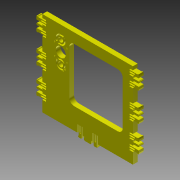
# Autodesk Inventor part: sideB
Saved by Autodesk Inventor 2012 SP1 (Build 160190100, 190)
## iProperties
Created: 2011-10-14
Part Number: sideB
Document SubType Name: Modeling
Designer: cramera
Density: 0.952 g/cm^3
Material: High Density Polyethylene
Mass: 347.048 g
Surface Area: 1035.52 cm^2
Volume: 364.546 cm^3
Autodesk Inventor part; units mm, degrees
ref_plane "YZ Plane" through (0, 0, 0) normal (1, 0, 0) x (0, 1, 0)
ref_plane "XZ Plane" through (0, 0, 0) normal (0, 1, 0) x (-1, 0, 0)
ref_plane "XY Plane" through (0, 0, 0) normal (0, 0, 1) x (1, 0, 0)
derived "skeleton.ipt"
sketch "DRILL-THROUGH" plane through (0, 0, 0) normal (0, 0, 1) x (1, 0, 0)
  arc A0 (221.6732, 527.9859) -> (220.0857, 526.3984) centre (221.6732, 526.3984) ccw
  arc A1 (220.0857, 526.3984) -> (221.6732, 524.8109) centre (221.6732, 526.3984) ccw
  arc A2 (221.6732, 524.8109) -> (223.2607, 526.3984) centre (221.6732, 526.3984) ccw
  arc A3 (223.2607, 526.3984) -> (221.6732, 527.9859) centre (221.6732, 526.3984) ccw
  arc A4 (252.6612, 527.9859) -> (251.0737, 526.3984) centre (252.6612, 526.3984) ccw
  arc A5 (251.0737, 526.3984) -> (252.6612, 524.8109) centre (252.6612, 526.3984) ccw
  arc A6 (252.6612, 524.8109) -> (254.2487, 526.3984) centre (252.6612, 526.3984) ccw
  arc A7 (254.2487, 526.3984) -> (252.6612, 527.9859) centre (252.6612, 526.3984) ccw
  arc A8 (252.6612, 496.9979) -> (251.0737, 495.4104) centre (252.6612, 495.4104) ccw
  arc A9 (251.0737, 495.4104) -> (252.6612, 493.8229) centre (252.6612, 495.4104) ccw
  arc A10 (252.6612, 493.8229) -> (254.2487, 495.4104) centre (252.6612, 495.4104) ccw
  arc A11 (254.2487, 495.4104) -> (252.6612, 496.9979) centre (252.6612, 495.4104) ccw
  arc A12 (221.6732, 496.9979) -> (220.0857, 495.4104) centre (221.6732, 495.4104) ccw
  arc A13 (220.0857, 495.4104) -> (221.6732, 493.8229) centre (221.6732, 495.4104) ccw
  arc A14 (221.6732, 493.8229) -> (223.2607, 495.4104) centre (221.6732, 495.4104) ccw
  arc A15 (223.2607, 495.4104) -> (221.6732, 496.9979) centre (221.6732, 495.4104) ccw
  constraints: 32 point on circle, 16 centre point
sketch "POCKET_1-8" plane through (0, 0, 0) normal (0, 0, 1) x (1, 0, 0)
  arc A0 (256.4712, 495.4104) -> (252.6612, 499.2204) centre (252.6612, 495.4104) ccw
  arc A1 (221.6732, 499.2204) -> (217.8632, 495.4104) centre (221.6732, 495.4104) ccw
  arc A2 (217.8632, 495.4104) -> (221.6732, 491.6004) centre (221.6732, 495.4104) ccw
  arc A3 (221.6732, 491.6004) -> (225.4832, 495.4104) centre (221.6732, 495.4104) ccw
  arc A4 (225.4832, 495.4104) -> (221.6732, 499.2204) centre (221.6732, 495.4104) ccw
  arc A5 (252.6612, 530.2084) -> (248.8512, 526.3984) centre (252.6612, 526.3984) ccw
  arc A6 (248.8512, 526.3984) -> (252.6612, 522.5884) centre (252.6612, 526.3984) ccw
  arc A7 (252.6612, 522.5884) -> (256.4712, 526.3984) centre (252.6612, 526.3984) ccw
  arc A8 (256.4712, 526.3984) -> (252.6612, 530.2084) centre (252.6612, 526.3984) ccw
  arc A9 (221.6732, 530.2084) -> (217.8632, 526.3984) centre (221.6732, 526.3984) ccw
  arc A10 (217.8632, 526.3984) -> (221.6732, 522.5884) centre (221.6732, 526.3984) ccw
  arc A11 (221.6732, 522.5884) -> (225.4832, 526.3984) centre (221.6732, 526.3984) ccw
  arc A12 (225.4832, 526.3984) -> (221.6732, 530.2084) centre (221.6732, 526.3984) ccw
  arc A13 (252.6612, 499.2204) -> (248.8512, 495.4104) centre (252.6612, 495.4104) ccw
  arc A14 (248.8512, 495.4104) -> (252.6612, 491.6004) centre (252.6612, 495.4104) ccw
  arc A15 (252.6612, 491.6004) -> (256.4712, 495.4104) centre (252.6612, 495.4104) ccw
  constraints: 32 point on circle, 16 centre point
sketch "STOCK_12MM" plane through (0, 0, 0) normal (0, 0, 1) x (1, 0, 0)
  line L0 (457.2, 0) -> (457.2, 914.4)
  line L1 (457.2, 914.4) -> (0, 914.4)
  line L2 (0, 914.4) -> (0, 0)
  line L3 (457.2, 914.4) -> (457.2, 0)
  line L4 (0, 0) -> (457.2, 0)
  constraints: 10 end point
sketch "THROUGH-CUT" plane through (0, 0, 0) normal (0, 0, 1) x (1, 0, 0)
  line L0 (271.4572, 409.3044) -> (381.6297, 409.3044)
  arc A0 (381.6297, 409.3044) -> (394.3297, 422.0044) centre (381.6297, 422.0044) ccw
  line L1 (394.3297, 422.0044) -> (394.3297, 533.1294)
  arc A1 (394.3297, 533.1294) -> (381.6297, 545.8294) centre (381.6297, 533.1294) ccw
  line L2 (381.6297, 545.8294) -> (271.4572, 545.8294)
  arc A2 (271.4572, 545.8294) -> (258.7572, 533.1294) centre (271.4572, 533.1294) ccw
  line L3 (258.7572, 533.1294) -> (258.7572, 422.0044)
  arc A3 (258.7572, 422.0044) -> (271.4572, 409.3044) centre (271.4572, 422.0044) ccw
  circle A4 centre (237.1672, 510.9044) radius 12.7
  circle A5 centre (237.1672, 537.8919) radius 5.925
  circle A6 centre (237.1672, 483.9169) radius 5.925
  arc A7 (410.2047, 390.0639) -> (411.7922, 388.4764) centre (411.7922, 390.0639) ccw
  line L4 (410.2047, 390.0639) -> (410.2047, 390.1909)
  arc A8 (411.7922, 391.7784) -> (410.2047, 390.1909) centre (411.7922, 390.1909) ccw
  line L5 (411.7922, 391.7784) -> (423.3207, 391.7784)
  arc A9 (424.9082, 390.1909) -> (423.3207, 391.7784) centre (423.3207, 390.1909) ccw
  line L6 (424.9082, 390.1909) -> (424.9082, 390.0639)
  arc A10 (423.3207, 388.4764) -> (424.9082, 390.0639) centre (423.3207, 390.0639) ccw
  line L7 (423.3207, 388.4764) -> (411.7922, 388.4764)
  arc A11 (423.3207, 553.8304) -> (424.9082, 555.4179) centre (423.3207, 555.4179) ccw
  line L8 (424.9082, 555.4179) -> (424.9082, 555.5449)
  arc A12 (424.9082, 555.5449) -> (423.3207, 557.1324) centre (423.3207, 555.5449) ccw
  line L9 (423.3207, 557.1324) -> (411.7922, 557.1324)
  arc A13 (411.7922, 557.1324) -> (410.2047, 555.5449) centre (411.7922, 555.5449) ccw
  line L10 (410.2047, 555.5449) -> (410.2047, 555.4179)
  arc A14 (410.2047, 555.4179) -> (411.7922, 553.8304) centre (411.7922, 555.4179) ccw
  line L11 (411.7922, 553.8304) -> (423.3207, 553.8304)
  arc A15 (410.2047, 415.7179) -> (411.7922, 414.1304) centre (411.7922, 415.7179) ccw
  line L12 (411.7922, 414.1304) -> (423.3207, 414.1304)
  arc A16 (423.3207, 414.1304) -> (424.9082, 415.7179) centre (423.3207, 415.7179) ccw
  line L13 (424.9082, 415.7179) -> (424.9082, 415.8449)
  arc A17 (424.9082, 415.8449) -> (423.3207, 417.4324) centre (423.3207, 415.8449) ccw
  line L14 (423.3207, 417.4324) -> (411.7922, 417.4324)
  arc A18 (411.7922, 417.4324) -> (410.2047, 415.8449) centre (411.7922, 415.8449) ccw
  line L15 (410.2047, 415.8449) -> (410.2047, 415.7179)
  arc A19 (423.3207, 455.1514) -> (424.9082, 456.7389) centre (423.3207, 456.7389) ccw
  line L16 (423.3207, 455.1514) -> (411.7922, 455.1514)
  arc A20 (410.2047, 456.7389) -> (411.7922, 455.1514) centre (411.7922, 456.7389) ccw
  line L17 (410.2047, 456.7389) -> (410.2047, 456.8659)
  arc A21 (411.7922, 458.4534) -> (410.2047, 456.8659) centre (411.7922, 456.8659) ccw
  line L18 (411.7922, 458.4534) -> (423.3207, 458.4534)
  arc A22 (424.9082, 456.8659) -> (423.3207, 458.4534) centre (423.3207, 456.8659) ccw
  line L19 (424.9082, 456.8659) -> (424.9082, 456.7389)
  arc A23 (423.3207, 528.1764) -> (424.9082, 529.7639) centre (423.3207, 529.7639) ccw
  line L20 (423.3207, 528.1764) -> (411.7922, 528.1764)
  arc A24 (410.2047, 529.7639) -> (411.7922, 528.1764) centre (411.7922, 529.7639) ccw
  line L21 (410.2047, 529.7639) -> (410.2047, 529.8909)
  arc A25 (411.7922, 531.4784) -> (410.2047, 529.8909) centre (411.7922, 529.8909) ccw
  line L22 (411.7922, 531.4784) -> (423.3207, 531.4784)
  arc A26 (424.9082, 529.8909) -> (423.3207, 531.4784) centre (423.3207, 529.8909) ccw
  line L23 (424.9082, 529.8909) -> (424.9082, 529.7639)
  arc A27 (284.6017, 358.0885) -> (286.1892, 356.501) centre (286.1892, 358.0885) ccw
  line L24 (284.6017, 358.0885) -> (284.6017, 372.7919)
  arc A28 (286.1892, 374.3794) -> (284.6017, 372.7919) centre (286.1892, 372.7919) ccw
  line L25 (286.1892, 374.3794) -> (286.3162, 374.3794)
  arc A29 (287.9037, 372.7919) -> (286.3162, 374.3794) centre (286.3162, 372.7919) ccw
  line L26 (287.9037, 372.7919) -> (287.9037, 358.0885)
  arc A30 (286.3162, 356.501) -> (287.9037, 358.0885) centre (286.3162, 358.0885) ccw
  line L27 (286.3162, 356.501) -> (286.1892, 356.501)
  arc A31 (187.5388, 417.4324) -> (185.9513, 415.8449) centre (187.5388, 415.8449) ccw
  line L28 (187.5388, 417.4324) -> (199.0672, 417.4324)
  arc A32 (200.6547, 415.8449) -> (199.0672, 417.4324) centre (199.0672, 415.8449) ccw
  line L29 (200.6547, 415.8449) -> (200.6547, 415.7179)
  arc A33 (199.0672, 414.1304) -> (200.6547, 415.7179) centre (199.0672, 415.7179) ccw
  line L30 (199.0672, 414.1304) -> (187.5388, 414.1304)
  arc A34 (185.9513, 415.7179) -> (187.5388, 414.1304) centre (187.5388, 415.7179) ccw
  line L31 (185.9513, 415.7179) -> (185.9513, 415.8449)
  arc A35 (187.5388, 391.7784) -> (185.9513, 390.1909) centre (187.5388, 390.1909) ccw
  line L32 (185.9513, 390.1909) -> (185.9513, 390.0639)
  arc A36 (185.9513, 390.0639) -> (187.5388, 388.4764) centre (187.5388, 390.0639) ccw
  line L33 (187.5388, 388.4764) -> (199.0672, 388.4764)
  arc A37 (199.0672, 388.4764) -> (200.6547, 390.0639) centre (199.0672, 390.0639) ccw
  line L34 (200.6547, 390.0639) -> (200.6547, 390.1909)
  arc A38 (200.6547, 390.1909) -> (199.0672, 391.7784) centre (199.0672, 390.1909) ccw
  line L35 (199.0672, 391.7784) -> (187.5388, 391.7784)
  arc A39 (199.0672, 480.8054) -> (200.6547, 482.3929) centre (199.0672, 482.3929) ccw
  line L36 (199.0672, 480.8054) -> (187.5388, 480.8054)
  arc A40 (185.9513, 482.3929) -> (187.5388, 480.8054) centre (187.5388, 482.3929) ccw
  line L37 (185.9513, 482.3929) -> (185.9513, 482.5199)
  arc A41 (187.5388, 484.1074) -> (185.9513, 482.5199) centre (187.5388, 482.5199) ccw
  line L38 (187.5388, 484.1074) -> (199.0672, 484.1074)
  arc A42 (200.6547, 482.5199) -> (199.0672, 484.1074) centre (199.0672, 482.5199) ccw
  line L39 (200.6547, 482.5199) -> (200.6547, 482.3929)
  arc A43 (228.9556, 532.1229) -> (229.2542, 533.9529) centre (227.8331, 533.2454) ccw
  line L40 (228.9556, 532.1229) -> (227.4719, 530.6392)
  arc A44 (225.2268, 530.6392) -> (227.4719, 530.6392) centre (226.3494, 531.7617) ccw
  line L41 (225.2268, 530.6392) -> (225.155, 530.711)
  arc A45 (225.155, 532.9561) -> (225.155, 530.711) centre (226.2775, 531.8336) ccw
  line L42 (225.155, 532.9561) -> (225.8266, 533.6277)
  arc A46 (241.4314, 549.2325) -> (225.8266, 533.6277) centre (237.1672, 537.8919) ccw
  line L43 (241.4314, 549.2325) -> (242.103, 549.9041)
  arc A47 (244.3481, 549.9041) -> (242.103, 549.9041) centre (243.2256, 548.7816) ccw
  line L44 (244.3481, 549.9041) -> (244.4199, 549.8323)
  arc A48 (244.4199, 547.5872) -> (244.4199, 549.8323) centre (243.2974, 548.7098) ccw
  line L45 (244.4199, 547.5872) -> (242.9362, 546.1035)
  arc A49 (241.1063, 545.8049) -> (242.9362, 546.1035) centre (241.8137, 547.226) ccw
  arc A50 (241.1063, 545.8049) -> (229.2542, 533.9529) centre (237.1672, 537.8919) ccw
  arc A51 (322.9557, 358.0885) -> (324.5432, 356.501) centre (324.5432, 358.0885) ccw
  line L46 (324.5432, 356.501) -> (324.6702, 356.501)
  arc A52 (324.6702, 356.501) -> (326.2577, 358.0885) centre (324.6702, 358.0885) ccw
  line L47 (326.2577, 358.0885) -> (326.2577, 372.7919)
  arc A53 (326.2577, 372.7919) -> (324.6702, 374.3794) centre (324.6702, 372.7919) ccw
  line L48 (324.6702, 374.3794) -> (324.5432, 374.3794)
  arc A54 (324.5432, 374.3794) -> (322.9557, 372.7919) centre (324.5432, 372.7919) ccw
  line L49 (322.9557, 372.7919) -> (322.9557, 358.0885)
  arc A55 (248.5078, 479.6527) -> (232.9031, 495.2575) centre (237.1672, 483.9169) ccw
  line L50 (232.9031, 495.2575) -> (232.2314, 495.9291)
  arc A56 (232.2314, 495.9291) -> (229.9864, 495.9291) centre (231.1089, 494.8066) ccw
  line L51 (229.9864, 495.9291) -> (229.9145, 495.8573)
  arc A57 (229.9145, 495.8573) -> (229.9145, 493.6122) centre (231.0371, 494.7348) ccw
  line L52 (229.9145, 493.6122) -> (231.3982, 492.1285)
  arc A58 (231.3982, 492.1285) -> (233.2282, 491.8299) centre (232.5208, 493.251) ccw
  arc A59 (245.0802, 479.9779) -> (233.2282, 491.8299) centre (237.1672, 483.9169) ccw
  arc A60 (245.0802, 479.9779) -> (245.3789, 478.1479) centre (246.5014, 479.2704) ccw
  line L53 (245.3789, 478.1479) -> (246.8626, 476.6642)
  arc A61 (246.8626, 476.6642) -> (249.1076, 476.6642) centre (247.9851, 477.7867) ccw
  line L54 (249.1076, 476.6642) -> (249.1795, 476.736)
  arc A62 (249.1795, 476.736) -> (249.1795, 478.9811) centre (248.0569, 477.8586) ccw
  line L55 (249.1795, 478.9811) -> (248.5078, 479.6527)
  arc A63 (199.0672, 528.1764) -> (200.6547, 529.7639) centre (199.0672, 529.7639) ccw
  line L56 (200.6547, 529.7639) -> (200.6547, 529.8909)
  arc A64 (200.6547, 529.8909) -> (199.0672, 531.4784) centre (199.0672, 529.8909) ccw
  line L57 (199.0672, 531.4784) -> (187.5388, 531.4784)
  arc A65 (187.5388, 531.4784) -> (185.9513, 529.8909) centre (187.5388, 529.8909) ccw
  line L58 (185.9513, 529.8909) -> (185.9513, 529.7639)
  arc A66 (185.9513, 529.7639) -> (187.5388, 528.1764) centre (187.5388, 529.7639) ccw
  line L59 (187.5388, 528.1764) -> (199.0672, 528.1764)
  arc A67 (423.3207, 480.8054) -> (424.9082, 482.3929) centre (423.3207, 482.3929) ccw
  line L60 (424.9082, 482.3929) -> (424.9082, 482.5199)
  arc A68 (424.9082, 482.5199) -> (423.3207, 484.1074) centre (423.3207, 482.5199) ccw
  line L61 (423.3207, 484.1074) -> (411.7922, 484.1074)
  arc A69 (411.7922, 484.1074) -> (410.2047, 482.5199) centre (411.7922, 482.5199) ccw
  line L62 (410.2047, 482.5199) -> (410.2047, 482.3929)
  arc A70 (410.2047, 482.3929) -> (411.7922, 480.8054) centre (411.7922, 482.3929) ccw
  line L63 (411.7922, 480.8054) -> (423.3207, 480.8054)
  arc A71 (187.5388, 458.4534) -> (185.9513, 456.8659) centre (187.5388, 456.8659) ccw
  line L64 (185.9513, 456.8659) -> (185.9513, 456.7389)
  arc A72 (185.9513, 456.7389) -> (187.5388, 455.1514) centre (187.5388, 456.7389) ccw
  line L65 (187.5388, 455.1514) -> (199.0616, 455.1514)
  arc A73 (199.0616, 455.1514) -> (200.6491, 456.7389) centre (199.0616, 456.7389) ccw
  line L66 (200.6491, 456.7389) -> (200.6547, 456.8659)
  arc A74 (200.6547, 456.8659) -> (199.0672, 458.4534) centre (199.0672, 456.8659) ccw
  line L67 (199.0672, 458.4534) -> (187.5388, 458.4534)
  arc A75 (225.8266, 488.1811) -> (241.4314, 472.5763) centre (237.1672, 483.9169) ccw
  line L68 (241.4314, 472.5763) -> (242.103, 471.9047)
  arc A76 (242.103, 471.9047) -> (244.3481, 471.9047) centre (243.2256, 473.0272) ccw
  line L69 (244.3481, 471.9047) -> (244.4199, 471.9765)
  arc A77 (244.4199, 471.9765) -> (244.4199, 474.2216) centre (243.2974, 473.099) ccw
  line L70 (244.4199, 474.2216) -> (242.9362, 475.7053)
  arc A78 (242.9362, 475.7053) -> (241.1063, 476.0039) centre (241.8137, 474.5827) ccw
  arc A79 (229.2542, 487.8559) -> (241.1063, 476.0039) centre (237.1672, 483.9169) ccw
  arc A80 (229.2542, 487.8559) -> (228.9556, 489.6859) centre (227.8331, 488.5634) ccw
  line L71 (228.9556, 489.6859) -> (227.4719, 491.1696)
  arc A81 (227.4719, 491.1696) -> (225.2268, 491.1696) centre (226.3494, 490.0471) ccw
  line L72 (225.2268, 491.1696) -> (225.155, 491.0978)
  arc A82 (225.155, 491.0978) -> (225.155, 488.8527) centre (226.2775, 489.9752) ccw
  line L73 (225.155, 488.8527) -> (225.8266, 488.1811)
  arc A83 (199.0672, 553.8304) -> (200.6547, 555.4179) centre (199.0672, 555.4179) ccw
  line L74 (199.0672, 553.8304) -> (187.5388, 553.8304)
  arc A84 (185.9513, 555.4179) -> (187.5388, 553.8304) centre (187.5388, 555.4179) ccw
  line L75 (185.9513, 555.4179) -> (185.9513, 555.5449)
  arc A85 (187.5388, 557.1324) -> (185.9513, 555.5449) centre (187.5388, 555.5449) ccw
  line L76 (187.5388, 557.1324) -> (199.0672, 557.1324)
  arc A86 (200.6547, 555.5449) -> (199.0672, 557.1324) centre (199.0672, 555.5449) ccw
  line L77 (200.6547, 555.5449) -> (200.6547, 555.4179)
  arc A87 (232.9031, 526.5513) -> (248.5078, 542.1561) centre (237.1672, 537.8919) ccw
  line L78 (232.9031, 526.5513) -> (232.2314, 525.8797)
  arc A88 (229.9864, 525.8797) -> (232.2314, 525.8797) centre (231.1089, 527.0022) ccw
  line L79 (229.9864, 525.8797) -> (229.9145, 525.9515)
  arc A89 (229.9145, 528.1966) -> (229.9145, 525.9515) centre (231.0371, 527.074) ccw
  line L80 (229.9145, 528.1966) -> (231.3982, 529.6803)
  arc A90 (233.2282, 529.9789) -> (231.3982, 529.6803) centre (232.5208, 528.5577) ccw
  arc A91 (233.2282, 529.9789) -> (245.0802, 541.8309) centre (237.1672, 537.8919) ccw
  arc A92 (245.3789, 543.6609) -> (245.0802, 541.8309) centre (246.5014, 542.5384) ccw
  line L81 (245.3789, 543.6609) -> (246.8626, 545.1446)
  arc A93 (249.1076, 545.1446) -> (246.8626, 545.1446) centre (247.9851, 544.0221) ccw
  line L82 (249.1076, 545.1446) -> (249.1795, 545.0728)
  arc A94 (249.1795, 542.8277) -> (249.1795, 545.0728) centre (248.0569, 543.9502) ccw
  line L83 (249.1795, 542.8277) -> (248.5078, 542.1561)
  arc A95 (288.3482, 346.4394) -> (289.9357, 348.0269) centre (288.3482, 348.0269) ccw
  line L84 (289.9357, 348.0269) -> (289.9357, 372.7919)
  arc A96 (291.5232, 374.3794) -> (289.9357, 372.7919) centre (291.5232, 372.7919) ccw
  line L85 (291.5232, 374.3794) -> (291.6502, 374.3794)
  arc A97 (293.2377, 372.7919) -> (291.6502, 374.3794) centre (291.6502, 372.7919) ccw
  line L86 (293.2377, 372.7919) -> (293.2377, 355.3294)
  line L87 (293.2377, 355.3294) -> (294.2947, 355.3294)
  arc A98 (296.5397, 353.0843) -> (294.2947, 355.3294) centre (295.4172, 354.2069) ccw
  line L88 (296.5397, 353.0843) -> (296.5397, 348.0269)
  line L89 (296.5397, 348.0269) -> (298.1272, 346.4394)
  line L90 (298.1272, 346.4394) -> (312.7322, 346.4394)
  line L91 (312.7322, 346.4394) -> (314.3197, 348.0269)
  line L92 (314.3197, 348.0269) -> (314.3197, 353.0843)
  arc A99 (316.5648, 355.3294) -> (314.3197, 353.0843) centre (315.4423, 354.2069) ccw
  line L93 (316.5648, 355.3294) -> (317.6217, 355.3294)
  line L94 (317.6217, 355.3294) -> (317.6217, 372.7919)
  arc A100 (319.2092, 374.3794) -> (317.6217, 372.7919) centre (319.2092, 372.7919) ccw
  line L95 (319.2092, 374.3794) -> (319.3362, 374.3794)
  arc A101 (320.9237, 372.7919) -> (319.3362, 374.3794) centre (319.3362, 372.7919) ccw
  line L96 (320.9237, 372.7919) -> (320.9237, 348.0269)
  arc A102 (320.9237, 348.0269) -> (322.509, 346.4394) centre (322.5112, 348.0269) ccw
  line L97 (322.509, 346.4394) -> (326.2142, 346.4394)
  line L98 (326.2142, 346.4394) -> (329.8137, 347.2615)
  line L99 (329.8137, 347.2615) -> (329.8137, 348.9794)
  line L100 (329.8137, 348.9794) -> (328.2897, 350.2494)
  line L101 (328.2897, 350.2494) -> (328.2897, 352.8767)
  line L102 (328.2897, 352.8767) -> (328.2897, 372.7919)
  arc A103 (329.8772, 374.3794) -> (328.2897, 372.7919) centre (329.8772, 372.7919) ccw
  line L103 (329.8772, 374.3794) -> (330.0042, 374.3794)
  arc A104 (331.5917, 372.7919) -> (330.0042, 374.3794) centre (330.0042, 372.7919) ccw
  line L104 (331.5917, 372.7919) -> (331.5917, 355.3294)
  line L105 (331.5917, 355.3294) -> (420.1107, 355.3294)
  line L106 (420.1107, 355.3294) -> (420.1107, 383.1424)
  line L107 (420.1107, 383.1424) -> (412.1732, 383.1424)
  arc A105 (410.5857, 384.7299) -> (412.1732, 383.1424) centre (412.1732, 384.7299) ccw
  line L108 (410.5857, 384.7299) -> (410.5857, 384.8569)
  arc A106 (412.1732, 386.4444) -> (410.5857, 384.8569) centre (412.1732, 384.8569) ccw
  line L109 (412.1732, 386.4444) -> (428.9135, 386.4444)
  line L110 (428.9135, 386.4444) -> (431.5407, 386.4444)
  line L111 (431.5407, 386.4444) -> (432.8107, 384.9204)
  line L112 (432.8107, 384.9204) -> (434.5287, 384.9204)
  line L113 (434.5287, 384.9204) -> (435.3507, 388.52)
  line L114 (435.3507, 388.52) -> (435.3507, 392.2251)
  arc A107 (435.3507, 392.2251) -> (433.7632, 393.8104) centre (433.7632, 392.2229) ccw
  line L115 (433.7632, 393.8104) -> (412.1732, 393.8104)
  arc A108 (410.5857, 395.3979) -> (412.1732, 393.8104) centre (412.1732, 395.3979) ccw
  line L116 (410.5857, 395.3979) -> (410.5857, 395.5249)
  arc A109 (412.1732, 397.1124) -> (410.5857, 395.5249) centre (412.1732, 395.5249) ccw
  line L117 (412.1732, 397.1124) -> (420.1107, 397.1124)
  line L118 (420.1107, 397.1124) -> (420.1107, 398.1693)
  arc A110 (422.3558, 400.4144) -> (420.1107, 398.1693) centre (421.2333, 399.2919) ccw
  line L119 (422.3558, 400.4144) -> (433.7632, 400.4144)
  line L120 (433.7632, 400.4144) -> (435.3507, 402.0019)
  line L121 (435.3507, 402.0019) -> (435.3507, 403.9069)
  line L122 (435.3507, 403.9069) -> (433.7632, 405.4944)
  line L123 (433.7632, 405.4944) -> (422.3558, 405.4944)
  arc A111 (420.1107, 407.7395) -> (422.3558, 405.4944) centre (421.2333, 406.6169) ccw
  line L124 (420.1107, 407.7395) -> (420.1107, 408.7964)
  line L125 (420.1107, 408.7964) -> (412.1732, 408.7964)
  arc A112 (410.5857, 410.3839) -> (412.1732, 408.7964) centre (412.1732, 410.3839) ccw
  line L126 (410.5857, 410.3839) -> (410.5857, 410.5109)
  arc A113 (412.1732, 412.0984) -> (410.5857, 410.5109) centre (412.1732, 410.5109) ccw
  line L127 (412.1732, 412.0984) -> (433.7632, 412.0984)
  arc A114 (433.7632, 412.0984) -> (435.3507, 413.6859) centre (433.7632, 413.6859) ccw
  line L128 (435.3507, 413.6859) -> (435.3507, 417.3888)
  line L129 (435.3507, 417.3888) -> (434.5287, 420.9884)
  line L130 (434.5287, 420.9884) -> (432.8107, 420.9884)
  line L131 (432.8107, 420.9884) -> (431.5407, 419.4644)
  line L132 (431.5407, 419.4644) -> (428.9135, 419.4644)
  line L133 (428.9135, 419.4644) -> (412.1732, 419.4644)
  arc A115 (410.5857, 421.0519) -> (412.1732, 419.4644) centre (412.1732, 421.0519) ccw
  line L134 (410.5857, 421.0519) -> (410.5857, 421.1789)
  arc A116 (412.1732, 422.7664) -> (410.5857, 421.1789) centre (412.1732, 421.1789) ccw
  line L135 (412.1732, 422.7664) -> (420.1107, 422.7664)
  line L136 (420.1107, 422.7664) -> (420.1107, 449.8174)
  line L137 (420.1107, 449.8174) -> (412.1732, 449.8174)
  arc A117 (410.5857, 451.4049) -> (412.1732, 449.8174) centre (412.1732, 451.4049) ccw
  line L138 (410.5857, 451.4049) -> (410.5857, 451.5319)
  arc A118 (412.1732, 453.1194) -> (410.5857, 451.5319) centre (412.1732, 451.5319) ccw
  line L139 (412.1732, 453.1194) -> (428.9135, 453.1194)
  line L140 (428.9135, 453.1194) -> (431.5407, 453.1194)
  line L141 (431.5407, 453.1194) -> (432.8107, 451.5954)
  line L142 (432.8107, 451.5954) -> (434.5287, 451.5954)
  line L143 (434.5287, 451.5954) -> (435.3507, 455.195)
  line L144 (435.3507, 455.195) -> (435.3507, 458.9001)
  arc A119 (435.3507, 458.9001) -> (433.7632, 460.4854) centre (433.7632, 458.8979) ccw
  line L145 (433.7632, 460.4854) -> (412.1732, 460.4854)
  arc A120 (410.5857, 462.0729) -> (412.1732, 460.4854) centre (412.1732, 462.0729) ccw
  line L146 (410.5857, 462.0729) -> (410.5857, 462.1999)
  arc A121 (412.1732, 463.7874) -> (410.5857, 462.1999) centre (412.1732, 462.1999) ccw
  line L147 (412.1732, 463.7874) -> (420.1107, 463.7874)
  line L148 (420.1107, 463.7874) -> (420.1107, 464.8443)
  arc A122 (422.3558, 467.0894) -> (420.1107, 464.8443) centre (421.2333, 465.9669) ccw
  line L149 (422.3558, 467.0894) -> (433.7632, 467.0894)
  line L150 (433.7632, 467.0894) -> (435.3507, 468.6769)
  line L151 (435.3507, 468.6769) -> (435.3507, 470.5819)
  line L152 (435.3507, 470.5819) -> (433.7632, 472.1694)
  line L153 (433.7632, 472.1694) -> (422.3558, 472.1694)
  arc A123 (420.1107, 474.4145) -> (422.3558, 472.1694) centre (421.2333, 473.2919) ccw
  line L154 (420.1107, 474.4145) -> (420.1107, 475.4714)
  line L155 (420.1107, 475.4714) -> (412.1732, 475.4714)
  arc A124 (410.5857, 477.0589) -> (412.1732, 475.4714) centre (412.1732, 477.0589) ccw
  line L156 (410.5857, 477.0589) -> (410.5857, 477.1859)
  arc A125 (412.1732, 478.7734) -> (410.5857, 477.1859) centre (412.1732, 477.1859) ccw
  line L157 (412.1732, 478.7734) -> (433.7632, 478.7734)
  arc A126 (433.7632, 478.7734) -> (435.3507, 480.3609) centre (433.7632, 480.3609) ccw
  line L158 (435.3507, 480.3609) -> (435.3507, 484.0638)
  line L159 (435.3507, 484.0638) -> (434.5287, 487.6634)
  line L160 (434.5287, 487.6634) -> (432.8107, 487.6634)
  line L161 (432.8107, 487.6634) -> (431.5407, 486.1394)
  line L162 (431.5407, 486.1394) -> (428.9135, 486.1394)
  line L163 (428.9135, 486.1394) -> (412.1732, 486.1394)
  arc A127 (410.5857, 487.7269) -> (412.1732, 486.1394) centre (412.1732, 487.7269) ccw
  line L164 (410.5857, 487.7269) -> (410.5857, 487.8539)
  arc A128 (412.1732, 489.4414) -> (410.5857, 487.8539) centre (412.1732, 487.8539) ccw
  line L165 (412.1732, 489.4414) -> (420.1107, 489.4414)
  line L166 (420.1107, 489.4414) -> (420.1107, 522.8424)
  line L167 (420.1107, 522.8424) -> (412.1732, 522.8424)
  arc A129 (410.5857, 524.4299) -> (412.1732, 522.8424) centre (412.1732, 524.4299) ccw
  line L168 (410.5857, 524.4299) -> (410.5857, 524.5569)
  arc A130 (412.1732, 526.1444) -> (410.5857, 524.5569) centre (412.1732, 524.5569) ccw
  line L169 (412.1732, 526.1444) -> (428.9135, 526.1444)
  line L170 (428.9135, 526.1444) -> (431.5407, 526.1444)
  line L171 (431.5407, 526.1444) -> (432.8107, 524.6204)
  line L172 (432.8107, 524.6204) -> (434.5287, 524.6204)
  line L173 (434.5287, 524.6204) -> (435.3507, 528.22)
  line L174 (435.3507, 528.22) -> (435.3507, 531.9251)
  arc A131 (435.3507, 531.9251) -> (433.7632, 533.5104) centre (433.7632, 531.9229) ccw
  line L175 (433.7632, 533.5104) -> (412.1732, 533.5104)
  arc A132 (410.5857, 535.0979) -> (412.1732, 533.5104) centre (412.1732, 535.0979) ccw
  line L176 (410.5857, 535.0979) -> (410.5857, 535.2249)
  arc A133 (412.1732, 536.8124) -> (410.5857, 535.2249) centre (412.1732, 535.2249) ccw
  line L177 (412.1732, 536.8124) -> (420.1107, 536.8124)
  line L178 (420.1107, 536.8124) -> (420.1107, 537.8693)
  arc A134 (422.3558, 540.1144) -> (420.1107, 537.8693) centre (421.2333, 538.9919) ccw
  line L179 (422.3558, 540.1144) -> (433.7632, 540.1144)
  line L180 (433.7632, 540.1144) -> (435.3507, 541.7019)
  line L181 (435.3507, 541.7019) -> (435.3507, 543.6069)
  line L182 (435.3507, 543.6069) -> (433.7632, 545.1944)
  line L183 (433.7632, 545.1944) -> (422.3558, 545.1944)
  arc A135 (420.1107, 547.4395) -> (422.3558, 545.1944) centre (421.2333, 546.3169) ccw
  line L184 (420.1107, 547.4395) -> (420.1107, 548.4964)
  line L185 (420.1107, 548.4964) -> (412.1732, 548.4964)
  arc A136 (410.5857, 550.0839) -> (412.1732, 548.4964) centre (412.1732, 550.0839) ccw
  line L186 (410.5857, 550.0839) -> (410.5857, 550.2109)
  arc A137 (412.1732, 551.7984) -> (410.5857, 550.2109) centre (412.1732, 550.2109) ccw
  line L187 (412.1732, 551.7984) -> (433.7632, 551.7984)
  arc A138 (433.7632, 551.7984) -> (435.3507, 553.3859) centre (433.7632, 553.3859) ccw
  line L188 (435.3507, 553.3859) -> (435.3507, 557.0888)
  line L189 (435.3507, 557.0888) -> (434.5287, 560.6884)
  line L190 (434.5287, 560.6884) -> (432.8107, 560.6884)
  line L191 (432.8107, 560.6884) -> (431.5407, 559.1644)
  line L192 (431.5407, 559.1644) -> (428.9135, 559.1644)
  line L193 (428.9135, 559.1644) -> (412.1732, 559.1644)
  arc A139 (410.5857, 560.7519) -> (412.1732, 559.1644) centre (412.1732, 560.7519) ccw
  line L194 (410.5857, 560.7519) -> (410.5857, 560.8789)
  arc A140 (412.1732, 562.4664) -> (410.5857, 560.8789) centre (412.1732, 560.8789) ccw
  line L195 (412.1732, 562.4664) -> (420.1107, 562.4664)
  line L196 (420.1107, 562.4664) -> (420.1107, 571.2294)
  line L197 (420.1107, 571.2294) -> (190.7487, 571.2294)
  line L198 (190.7487, 571.2294) -> (190.7487, 562.4664)
  line L199 (190.7487, 562.4664) -> (198.6862, 562.4664)
  arc A141 (200.2737, 560.8789) -> (198.6862, 562.4664) centre (198.6862, 560.8789) ccw
  line L200 (200.2737, 560.8789) -> (200.2737, 560.7519)
  arc A142 (198.6862, 559.1644) -> (200.2737, 560.7519) centre (198.6862, 560.7519) ccw
  line L201 (198.6862, 559.1644) -> (181.946, 559.1644)
  line L202 (181.946, 559.1644) -> (179.3187, 559.1644)
  line L203 (179.3187, 559.1644) -> (178.0487, 560.6884)
  line L204 (178.0487, 560.6884) -> (176.3308, 560.6884)
  line L205 (176.3308, 560.6884) -> (175.5087, 557.0888)
  line L206 (175.5087, 557.0888) -> (175.5087, 553.3859)
  arc A143 (175.5087, 553.3859) -> (177.0962, 551.7984) centre (177.0962, 553.3859) ccw
  line L207 (177.0962, 551.7984) -> (198.6862, 551.7984)
  arc A144 (200.2737, 550.2109) -> (198.6862, 551.7984) centre (198.6862, 550.2109) ccw
  line L208 (200.2737, 550.2109) -> (200.2737, 550.0839)
  arc A145 (198.6862, 548.4964) -> (200.2737, 550.0839) centre (198.6862, 550.0839) ccw
  line L209 (198.6862, 548.4964) -> (190.7487, 548.4964)
  line L210 (190.7487, 548.4964) -> (190.7487, 547.4395)
  arc A146 (188.5037, 545.1944) -> (190.7487, 547.4395) centre (189.6262, 546.3169) ccw
  line L211 (188.5037, 545.1944) -> (177.0962, 545.1944)
  line L212 (177.0962, 545.1944) -> (175.5087, 543.6069)
  line L213 (175.5087, 543.6069) -> (175.5087, 541.7019)
  line L214 (175.5087, 541.7019) -> (177.0962, 540.1144)
  line L215 (177.0962, 540.1144) -> (188.5037, 540.1144)
  arc A147 (190.7487, 537.8693) -> (188.5037, 540.1144) centre (189.6262, 538.9919) ccw
  line L216 (190.7487, 537.8693) -> (190.7487, 536.8124)
  line L217 (190.7487, 536.8124) -> (198.6862, 536.8124)
  arc A148 (200.2737, 535.2249) -> (198.6862, 536.8124) centre (198.6862, 535.2249) ccw
  line L218 (200.2737, 535.2249) -> (200.2737, 535.0979)
  arc A149 (198.6862, 533.5104) -> (200.2737, 535.0979) centre (198.6862, 535.0979) ccw
  line L219 (198.6862, 533.5104) -> (177.0962, 533.5104)
  arc A150 (177.0962, 533.5104) -> (175.5087, 531.9251) centre (177.0962, 531.9229) ccw
  line L220 (175.5087, 531.9251) -> (175.5087, 528.22)
  line L221 (175.5087, 528.22) -> (176.3308, 524.6204)
  line L222 (176.3308, 524.6204) -> (178.0487, 524.6204)
  line L223 (178.0487, 524.6204) -> (179.3187, 526.1444)
  line L224 (179.3187, 526.1444) -> (181.946, 526.1444)
  line L225 (181.946, 526.1444) -> (198.6862, 526.1444)
  arc A151 (200.2737, 524.5569) -> (198.6862, 526.1444) centre (198.6862, 524.5569) ccw
  line L226 (200.2737, 524.5569) -> (200.2737, 524.4299)
  arc A152 (198.6862, 522.8424) -> (200.2737, 524.4299) centre (198.6862, 524.4299) ccw
  line L227 (198.6862, 522.8424) -> (190.7487, 522.8424)
  line L228 (190.7487, 522.8424) -> (190.7487, 489.4414)
  line L229 (190.7487, 489.4414) -> (198.6862, 489.4414)
  arc A153 (200.2737, 487.8539) -> (198.6862, 489.4414) centre (198.6862, 487.8539) ccw
  line L230 (200.2737, 487.8539) -> (200.2737, 487.7269)
  arc A154 (198.6862, 486.1394) -> (200.2737, 487.7269) centre (198.6862, 487.7269) ccw
  line L231 (198.6862, 486.1394) -> (181.946, 486.1394)
  line L232 (181.946, 486.1394) -> (179.3187, 486.1394)
  line L233 (179.3187, 486.1394) -> (178.0487, 487.6634)
  line L234 (178.0487, 487.6634) -> (176.3308, 487.6634)
  line L235 (176.3308, 487.6634) -> (175.5087, 484.0638)
  line L236 (175.5087, 484.0638) -> (175.5087, 480.3609)
  arc A155 (175.5087, 480.3609) -> (177.0962, 478.7734) centre (177.0962, 480.3609) ccw
  line L237 (177.0962, 478.7734) -> (198.6862, 478.7734)
  arc A156 (200.2737, 477.1859) -> (198.6862, 478.7734) centre (198.6862, 477.1859) ccw
  line L238 (200.2737, 477.1859) -> (200.2737, 477.0589)
  arc A157 (198.6862, 475.4714) -> (200.2737, 477.0589) centre (198.6862, 477.0589) ccw
  line L239 (198.6862, 475.4714) -> (190.7487, 475.4714)
  line L240 (190.7487, 475.4714) -> (190.7487, 474.4145)
  arc A158 (188.5037, 472.1694) -> (190.7487, 474.4145) centre (189.6262, 473.2919) ccw
  line L241 (188.5037, 472.1694) -> (177.0962, 472.1694)
  line L242 (177.0962, 472.1694) -> (175.5087, 470.5819)
  line L243 (175.5087, 470.5819) -> (175.5087, 468.6769)
  line L244 (175.5087, 468.6769) -> (177.0962, 467.0894)
  line L245 (177.0962, 467.0894) -> (188.5037, 467.0894)
  arc A159 (190.7487, 464.8443) -> (188.5037, 467.0894) centre (189.6262, 465.9669) ccw
  line L246 (190.7487, 464.8443) -> (190.7487, 463.7874)
  line L247 (190.7487, 463.7874) -> (198.6862, 463.7874)
  arc A160 (200.2737, 462.1999) -> (198.6862, 463.7874) centre (198.6862, 462.1999) ccw
  line L248 (200.2737, 462.1999) -> (200.2737, 462.0729)
  arc A161 (198.6862, 460.4854) -> (200.2737, 462.0729) centre (198.6862, 462.0729) ccw
  line L249 (198.6862, 460.4854) -> (177.0962, 460.4854)
  arc A162 (177.0962, 460.4854) -> (175.5087, 458.9001) centre (177.0962, 458.8979) ccw
  line L250 (175.5087, 458.9001) -> (175.5087, 455.195)
  line L251 (175.5087, 455.195) -> (176.3308, 451.5954)
  line L252 (176.3308, 451.5954) -> (178.0487, 451.5954)
  line L253 (178.0487, 451.5954) -> (179.3187, 453.1194)
  line L254 (179.3187, 453.1194) -> (181.946, 453.1194)
  line L255 (181.946, 453.1194) -> (198.6862, 453.1194)
  arc A163 (200.2737, 451.5319) -> (198.6862, 453.1194) centre (198.6862, 451.5319) ccw
  line L256 (200.2737, 451.5319) -> (200.2737, 451.4049)
  arc A164 (198.6862, 449.8174) -> (200.2737, 451.4049) centre (198.6862, 451.4049) ccw
  line L257 (198.6862, 449.8174) -> (190.7487, 449.8174)
  line L258 (190.7487, 449.8174) -> (190.7487, 422.7664)
  line L259 (190.7487, 422.7664) -> (198.6862, 422.7664)
  arc A165 (200.2737, 421.1789) -> (198.6862, 422.7664) centre (198.6862, 421.1789) ccw
  line L260 (200.2737, 421.1789) -> (200.2737, 421.0519)
  arc A166 (198.6862, 419.4644) -> (200.2737, 421.0519) centre (198.6862, 421.0519) ccw
  line L261 (198.6862, 419.4644) -> (181.946, 419.4644)
  line L262 (181.946, 419.4644) -> (179.3187, 419.4644)
  line L263 (179.3187, 419.4644) -> (178.0487, 420.9884)
  line L264 (178.0487, 420.9884) -> (176.3308, 420.9884)
  line L265 (176.3308, 420.9884) -> (175.5087, 417.3888)
  line L266 (175.5087, 417.3888) -> (175.5087, 413.6859)
  arc A167 (175.5087, 413.6859) -> (177.0962, 412.0984) centre (177.0962, 413.6859) ccw
  line L267 (177.0962, 412.0984) -> (198.6862, 412.0984)
  arc A168 (200.2737, 410.5109) -> (198.6862, 412.0984) centre (198.6862, 410.5109) ccw
  line L268 (200.2737, 410.5109) -> (200.2737, 410.3839)
  arc A169 (198.6862, 408.7964) -> (200.2737, 410.3839) centre (198.6862, 410.3839) ccw
  line L269 (198.6862, 408.7964) -> (190.7487, 408.7964)
  line L270 (190.7487, 408.7964) -> (190.7487, 407.7395)
  arc A170 (188.5037, 405.4944) -> (190.7487, 407.7395) centre (189.6262, 406.6169) ccw
  line L271 (188.5037, 405.4944) -> (177.0962, 405.4944)
  line L272 (177.0962, 405.4944) -> (175.5087, 403.9069)
  line L273 (175.5087, 403.9069) -> (175.5087, 402.0019)
  line L274 (175.5087, 402.0019) -> (177.0962, 400.4144)
  line L275 (177.0962, 400.4144) -> (188.5037, 400.4144)
  arc A171 (190.7487, 398.1693) -> (188.5037, 400.4144) centre (189.6262, 399.2919) ccw
  line L276 (190.7487, 398.1693) -> (190.7487, 397.1124)
  line L277 (190.7487, 397.1124) -> (198.6862, 397.1124)
  arc A172 (200.2737, 395.5249) -> (198.6862, 397.1124) centre (198.6862, 395.5249) ccw
  line L278 (200.2737, 395.5249) -> (200.2737, 395.3979)
  arc A173 (198.6862, 393.8104) -> (200.2737, 395.3979) centre (198.6862, 395.3979) ccw
  line L279 (198.6862, 393.8104) -> (177.0962, 393.8104)
  arc A174 (177.0962, 393.8104) -> (175.5087, 392.2251) centre (177.0962, 392.2229) ccw
  line L280 (175.5087, 392.2251) -> (175.5087, 388.52)
  line L281 (175.5087, 388.52) -> (176.3308, 384.9204)
  line L282 (176.3308, 384.9204) -> (178.0487, 384.9204)
  line L283 (178.0487, 384.9204) -> (179.3187, 386.4444)
  line L284 (179.3187, 386.4444) -> (181.946, 386.4444)
  line L285 (181.946, 386.4444) -> (198.6862, 386.4444)
  arc A175 (200.2737, 384.8569) -> (198.6862, 386.4444) centre (198.6862, 384.8569) ccw
  line L286 (200.2737, 384.8569) -> (200.2737, 384.7299)
  arc A176 (198.6862, 383.1424) -> (200.2737, 384.7299) centre (198.6862, 384.7299) ccw
  line L287 (198.6862, 383.1424) -> (190.7487, 383.1424)
  line L288 (190.7487, 383.1424) -> (190.7487, 355.3294)
  line L289 (190.7487, 355.3294) -> (279.2677, 355.3294)
  line L290 (279.2677, 355.3294) -> (279.2677, 372.7919)
  arc A177 (280.8552, 374.3794) -> (279.2677, 372.7919) centre (280.8552, 372.7919) ccw
  line L291 (280.8552, 374.3794) -> (280.9822, 374.3794)
  arc A178 (282.5697, 372.7919) -> (280.9822, 374.3794) centre (280.9822, 372.7919) ccw
  line L292 (282.5697, 372.7919) -> (282.5697, 352.8767)
  line L293 (282.5697, 352.8767) -> (282.5697, 350.2494)
  line L294 (282.5697, 350.2494) -> (281.0457, 348.9794)
  line L295 (281.0457, 348.9794) -> (281.0457, 347.2615)
  line L296 (281.0457, 347.2615) -> (284.6453, 346.4394)
  line L297 (284.6453, 346.4394) -> (288.3482, 346.4394)
  dimension "d7" = 11.85
  dimension "d8" = 11.85
  dimension "d9" = 53.975
  constraints: 596 end point, 352 point on circle, 179 centre point
  measures "d7" diameter of A5
  measures "d8" diameter of A6
  measures "d9" distance of A6.centre A5.centre
extrude "Extrusion1" add sketch "THROUGH-CUT" along normal blind 12
extrude "Extrusion2" cut sketch "POCKET_1-8" along normal blind 3.175
extrude "Extrusion3" cut sketch "DRILL-THROUGH" along normal through all
equation "\"d8\" = d7"
equation "\"d1\" = StockThickness"
equation "\"StockThickness\" = 12"
body "Solid1"
